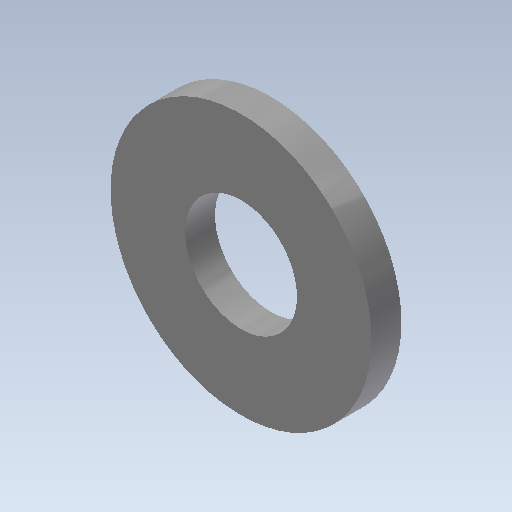
# Autodesk Inventor part: Washer 8 ID
Saved by Autodesk Inventor 2020 (Build 240168000, 168)
## iProperties
Created: 2014-11-29
Part Number: Washer 8 ID
Material: Steel
Document SubType Name: Modeling
Designer: Nemo
Density: 7.85 g/cm^3
Appearance: Steel
Author: Nemo
Autodesk Inventor part; units mm, degrees
ref_plane "YZ Plane" through (0, 0, 0) normal (1, 0, 0) x (0, 1, 0)
ref_plane "XZ Plane" through (0, 0, 0) normal (0, 1, 0) x (-1, 0, 0)
ref_plane "XY Plane" through (0, 0, 0) normal (0, 0, 1) x (1, 0, 0)
sketch "Sketch1" plane through (0, 0, 0) normal (0, 0, 1) x (1, 0, 0)
  circle A0 centre (0, 0) radius 2.3812
  circle A1 centre (0, 0) radius 5.5563
  dimension "d0" = 4.7625
  dimension "d1" = 11.1125
  constraints: 2 centre point, 2 coincident
  measures "d0" diameter of A0
  measures "d1" diameter of A1
extrude "Extrusion1" add sketch "Sketch1" along normal blind 1.27
body "Solid1"
